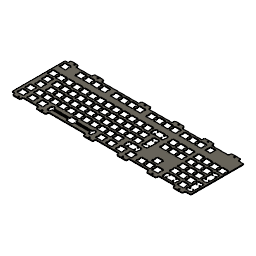
Plate (Autodesk Fusion 360 design; units mm, degrees)
part number: 2026-01-24-23-38-07-205
Autodesk Fusion 360 part; units mm, degrees
(part 1 of 3)
sketch "Sketch2" plane through (0, 0, 0) normal (0, 0, 1) x (1, 0, 0)
  line L0 (432.82, 128.316) -> (432.82, 0.1902)
  line L1 (0.0951, 0.1902) -> (0.0951, 128.316)
  line L2 (126.263, 19.0169) -> (126.263, 18.0165)
  line L3 (126.263, 18.0165) -> (125.462, 18.0165)
  line L4 (125.462, 18.0165) -> (125.462, 14.9173)
  line L5 (125.462, 14.9173) -> (126.263, 14.9173)
  line L6 (126.263, 14.9173) -> (126.263, 14.3164)
  line L7 (126.263, 14.3164) -> (86.6373, 14.3164)
  line L8 (86.6373, 14.3164) -> (86.6373, 17.5466)
  line L9 (86.6373, 17.5466) -> (84.9119, 17.5466)
  line L10 (84.9119, 17.5466) -> (84.9119, 18.4671)
  line L11 (84.9119, 18.4671) -> (81.613, 18.4671)
  line L12 (81.613, 18.4671) -> (81.613, 17.5466)
  line L13 (81.613, 17.5466) -> (79.8876, 17.5466)
  line L14 (79.8876, 17.5466) -> (79.8876, 14.3164)
  line L15 (79.8876, 14.3164) -> (79.0621, 14.3164)
  line L16 (79.0621, 14.3164) -> (79.0621, 11.5163)
  line L17 (79.0621, 11.5163) -> (79.8876, 11.5163)
  line L18 (79.8876, 11.5163) -> (79.8876, 5.2462)
  line L19 (79.8876, 5.2462) -> (81.613, 5.2462)
  line L20 (81.613, 5.2462) -> (81.613, 4.2664)
  line L21 (81.613, 4.2664) -> (84.9119, 4.2664)
  line L22 (84.9119, 4.2664) -> (84.9119, 5.2462)
  line L23 (84.9119, 5.2462) -> (86.6373, 5.2462)
  line L24 (86.6373, 5.2462) -> (86.6373, 9.7166)
  line L25 (86.6373, 9.7166) -> (126.263, 9.7166)
  line L26 (126.263, 9.7166) -> (126.263, 9.1171)
  line L27 (126.263, 9.1171) -> (125.462, 9.1171)
  line L28 (125.462, 9.1171) -> (125.462, 6.0165)
  line L29 (125.462, 6.0165) -> (126.263, 6.0165)
  line L30 (126.263, 6.0165) -> (126.263, 5.0161)
  line L31 (126.263, 5.0161) -> (140.262, 5.0161)
  line L32 (140.262, 5.0161) -> (140.262, 6.0165)
  line L33 (140.262, 6.0165) -> (141.063, 6.0165)
  line L34 (141.063, 6.0165) -> (141.063, 9.1171)
  line L35 (141.063, 9.1171) -> (140.262, 9.1171)
  line L36 (140.262, 9.1171) -> (140.262, 9.7166)
  line L37 (140.262, 9.7166) -> (179.888, 9.7166)
  line L38 (179.888, 9.7166) -> (179.888, 5.2462)
  line L39 (179.888, 5.2462) -> (181.613, 5.2462)
  line L40 (181.613, 5.2462) -> (181.613, 4.2664)
  line L41 (181.613, 4.2664) -> (184.912, 4.2664)
  line L42 (184.912, 4.2664) -> (184.912, 5.2462)
  line L43 (184.912, 5.2462) -> (186.637, 5.2462)
  line L44 (186.637, 5.2462) -> (186.637, 11.5163)
  line L45 (186.637, 11.5163) -> (187.463, 11.5163)
  line L46 (187.463, 11.5163) -> (187.463, 14.3164)
  line L47 (187.463, 14.3164) -> (186.637, 14.3164)
  line L48 (186.637, 14.3164) -> (186.637, 17.5466)
  line L49 (186.637, 17.5466) -> (184.912, 17.5466)
  line L50 (184.912, 17.5466) -> (184.912, 18.4671)
  line L51 (184.912, 18.4671) -> (181.613, 18.4671)
  line L52 (181.613, 18.4671) -> (181.613, 17.5466)
  line L53 (181.613, 17.5466) -> (179.888, 17.5466)
  line L54 (179.888, 17.5466) -> (179.888, 14.3164)
  line L55 (179.888, 14.3164) -> (140.262, 14.3164)
  line L56 (140.262, 14.3164) -> (140.262, 14.9173)
  line L57 (140.262, 14.9173) -> (141.063, 14.9173)
  line L58 (141.063, 14.9173) -> (141.063, 18.0165)
  line L59 (141.063, 18.0165) -> (140.262, 18.0165)
  line L60 (140.262, 18.0165) -> (140.262, 19.0169)
  line L61 (140.262, 19.0169) -> (126.263, 19.0169)
  line L62 (366.769, 19.0169) -> (366.769, 18.0165)
  line L63 (366.769, 18.0165) -> (365.968, 18.0165)
  line L64 (365.968, 18.0165) -> (365.968, 14.9173)
  line L65 (365.968, 14.9173) -> (366.769, 14.9173)
  line L66 (366.769, 14.9173) -> (366.769, 14.3164)
  line L67 (366.769, 14.3164) -> (365.245, 14.3164)
  line L68 (365.245, 14.3164) -> (365.245, 17.5466)
  line L69 (365.245, 17.5466) -> (363.52, 17.5466)
  line L70 (363.52, 17.5466) -> (363.52, 18.4671)
  line L71 (363.52, 18.4671) -> (360.218, 18.4671)
  line L72 (360.218, 18.4671) -> (360.218, 17.5466)
  line L73 (360.218, 17.5466) -> (358.493, 17.5466)
  line L74 (358.493, 17.5466) -> (358.493, 14.3164)
  line L75 (358.493, 14.3164) -> (357.671, 14.3164)
  line L76 (357.671, 14.3164) -> (357.671, 11.5163)
  line L77 (357.671, 11.5163) -> (358.493, 11.5163)
  line L78 (358.493, 11.5163) -> (358.493, 5.2462)
  line L79 (358.493, 5.2462) -> (360.218, 5.2462)
  line L80 (360.218, 5.2462) -> (360.218, 4.2664)
  line L81 (360.218, 4.2664) -> (363.52, 4.2664)
  line L82 (363.52, 4.2664) -> (363.52, 5.2462)
  line L83 (363.52, 5.2462) -> (365.245, 5.2462)
  line L84 (365.245, 5.2462) -> (365.245, 9.7166)
  line L85 (365.245, 9.7166) -> (366.769, 9.7166)
  line L86 (366.769, 9.7166) -> (366.769, 9.1171)
  line L87 (366.769, 9.1171) -> (365.968, 9.1171)
  line L88 (365.968, 9.1171) -> (365.968, 6.0165)
  line L89 (365.968, 6.0165) -> (366.769, 6.0165)
  line L90 (366.769, 6.0165) -> (366.769, 5.0161)
  line L91 (366.769, 5.0161) -> (380.771, 5.0161)
  line L92 (380.771, 5.0161) -> (380.771, 6.0165)
  line L93 (380.771, 6.0165) -> (381.568, 6.0165)
  line L94 (381.568, 6.0165) -> (381.568, 9.1171)
  line L95 (381.568, 9.1171) -> (380.771, 9.1171)
  line L96 (380.771, 9.1171) -> (380.771, 9.7166)
  line L97 (380.771, 9.7166) -> (382.295, 9.7166)
  line L98 (382.295, 9.7166) -> (382.295, 5.2462)
  line L99 (382.295, 5.2462) -> (384.02, 5.2462)
  line L100 (384.02, 5.2462) -> (384.02, 4.2664)
  line L101 (384.02, 4.2664) -> (387.318, 4.2664)
  line L102 (387.318, 4.2664) -> (387.318, 5.2462)
  line L103 (387.318, 5.2462) -> (389.043, 5.2462)
  line L104 (389.043, 5.2462) -> (389.043, 11.5163)
  line L105 (389.043, 11.5163) -> (389.869, 11.5163)
  line L106 (389.869, 11.5163) -> (389.869, 14.3164)
  line L107 (389.869, 14.3164) -> (389.043, 14.3164)
  line L108 (389.043, 14.3164) -> (389.043, 17.5466)
  line L109 (389.043, 17.5466) -> (387.318, 17.5466)
  line L110 (387.318, 17.5466) -> (387.318, 18.4671)
  line L111 (387.318, 18.4671) -> (384.02, 18.4671)
  line L112 (384.02, 18.4671) -> (384.02, 17.5466)
  line L113 (384.02, 17.5466) -> (382.295, 17.5466)
  line L114 (382.295, 17.5466) -> (382.295, 14.3164)
  line L115 (382.295, 14.3164) -> (380.771, 14.3164)
  line L116 (380.771, 14.3164) -> (380.771, 14.9173)
  line L117 (380.771, 14.9173) -> (381.568, 14.9173)
  line L118 (381.568, 14.9173) -> (381.568, 18.0165)
  line L119 (381.568, 18.0165) -> (380.771, 18.0165)
  line L120 (380.771, 18.0165) -> (380.771, 19.0169)
  line L121 (380.771, 19.0169) -> (366.769, 19.0169)
  line L122 (7.2003, 19.0169) -> (7.2003, 18.0165)
  line L123 (7.2003, 18.0165) -> (6.401, 18.0165)
  line L124 (6.401, 18.0165) -> (6.401, 14.9173)
  line L125 (6.401, 14.9173) -> (7.2003, 14.9173)
  line L126 (7.2003, 14.9173) -> (7.2003, 9.1171)
  line L127 (7.2003, 9.1171) -> (6.401, 9.1171)
  line L128 (6.401, 9.1171) -> (6.401, 6.0165)
  line L129 (6.401, 6.0165) -> (7.2003, 6.0165)
  line L130 (7.2003, 6.0165) -> (7.2003, 5.0161)
  line L131 (7.2003, 5.0161) -> (21.2011, 5.0161)
  line L132 (21.2011, 5.0161) -> (21.2011, 6.0165)
  line L133 (21.2011, 6.0165) -> (22.0004, 6.0165)
  line L134 (22.0004, 6.0165) -> (22.0004, 9.1171)
  line L135 (22.0004, 9.1171) -> (21.2011, 9.1171)
  line L136 (21.2011, 9.1171) -> (21.2011, 14.9173)
  line L137 (21.2011, 14.9173) -> (22.0004, 14.9173)
  line L138 (22.0004, 14.9173) -> (22.0004, 18.0165)
  line L139 (22.0004, 18.0165) -> (21.2011, 18.0165)
  line L140 (21.2011, 18.0165) -> (21.2011, 19.0169)
  line L141 (21.2011, 19.0169) -> (7.2003, 19.0169)
  line L142 (31.0128, 19.0169) -> (31.0128, 18.0165)
  line L143 (31.0128, 18.0165) -> (30.2121, 18.0165)
  line L144 (30.2121, 18.0165) -> (30.2121, 14.9173)
  line L145 (30.2121, 14.9173) -> (31.0128, 14.9173)
  line L146 (31.0128, 14.9173) -> (31.0128, 9.1171)
  line L147 (31.0128, 9.1171) -> (30.2121, 9.1171)
  line L148 (30.2121, 9.1171) -> (30.2121, 6.0165)
  line L149 (30.2121, 6.0165) -> (31.0128, 6.0165)
  line L150 (31.0128, 6.0165) -> (31.0128, 5.0161)
  line L151 (31.0128, 5.0161) -> (45.0123, 5.0161)
  line L152 (45.0123, 5.0161) -> (45.0123, 6.0165)
  line L153 (45.0123, 6.0165) -> (45.8128, 6.0165)
  line L154 (45.8128, 6.0165) -> (45.8128, 9.1171)
  line L155 (45.8128, 9.1171) -> (45.0123, 9.1171)
  line L156 (45.0123, 9.1171) -> (45.0123, 14.9173)
  line L157 (45.0123, 14.9173) -> (45.8128, 14.9173)
  line L158 (45.8128, 14.9173) -> (45.8128, 18.0165)
  line L159 (45.8128, 18.0165) -> (45.0123, 18.0165)
  line L160 (45.0123, 18.0165) -> (45.0123, 19.0169)
  line L161 (45.0123, 19.0169) -> (31.0128, 19.0169)
  line L162 (54.8252, 19.0169) -> (54.8252, 18.0165)
  line L163 (54.8252, 18.0165) -> (54.0262, 18.0165)
  line L164 (54.0262, 18.0165) -> (54.0262, 14.9173)
  line L165 (54.0262, 14.9173) -> (54.8252, 14.9173)
  line L166 (54.8252, 14.9173) -> (54.8252, 9.1171)
  line L167 (54.8252, 9.1171) -> (54.0262, 9.1171)
  line L168 (54.0262, 9.1171) -> (54.0262, 6.0165)
  line L169 (54.0262, 6.0165) -> (54.8252, 6.0165)
  line L170 (54.8252, 6.0165) -> (54.8252, 5.0161)
  line L171 (54.8252, 5.0161) -> (68.8262, 5.0161)
  line L172 (68.8262, 5.0161) -> (68.8262, 6.0165)
  line L173 (68.8262, 6.0165) -> (69.6253, 6.0165)
  line L174 (69.6253, 6.0165) -> (69.6253, 9.1171)
  line L175 (69.6253, 9.1171) -> (68.8262, 9.1171)
  line L176 (68.8262, 9.1171) -> (68.8262, 14.9173)
  line L177 (68.8262, 14.9173) -> (69.6253, 14.9173)
  line L178 (69.6253, 14.9173) -> (69.6253, 18.0165)
  line L179 (69.6253, 18.0165) -> (68.8262, 18.0165)
  line L180 (68.8262, 18.0165) -> (68.8262, 19.0169)
  line L181 (68.8262, 19.0169) -> (54.8252, 19.0169)
  line L182 (197.7, 19.0169) -> (197.7, 18.0165)
  line L183 (197.7, 18.0165) -> (196.901, 18.0165)
  line L184 (196.901, 18.0165) -> (196.901, 14.9173)
  line L185 (196.901, 14.9173) -> (197.7, 14.9173)
  line L186 (197.7, 14.9173) -> (197.7, 9.1171)
  line L187 (197.7, 9.1171) -> (196.901, 9.1171)
  line L188 (196.901, 9.1171) -> (196.901, 6.0165)
  line L189 (196.901, 6.0165) -> (197.7, 6.0165)
  line L190 (197.7, 6.0165) -> (197.7, 5.0161)
  line L191 (197.7, 5.0161) -> (211.701, 5.0161)
  line L192 (211.701, 5.0161) -> (211.701, 6.0165)
  line L193 (211.701, 6.0165) -> (212.5, 6.0165)
  line L194 (212.5, 6.0165) -> (212.5, 9.1171)
  line L195 (212.5, 9.1171) -> (211.701, 9.1171)
  line L196 (211.701, 9.1171) -> (211.701, 14.9173)
  line L197 (211.701, 14.9173) -> (212.5, 14.9173)
  line L198 (212.5, 14.9173) -> (212.5, 18.0165)
  line L199 (212.5, 18.0165) -> (211.701, 18.0165)
  line L200 (211.701, 18.0165) -> (211.701, 19.0169)
  line L201 (211.701, 19.0169) -> (197.7, 19.0169)
  line L202 (221.513, 19.0169) -> (221.513, 18.0165)
  line L203 (221.513, 18.0165) -> (220.712, 18.0165)
  line L204 (220.712, 18.0165) -> (220.712, 14.9173)
  line L205 (220.712, 14.9173) -> (221.513, 14.9173)
  line L206 (221.513, 14.9173) -> (221.513, 9.1171)
  line L207 (221.513, 9.1171) -> (220.712, 9.1171)
  line L208 (220.712, 9.1171) -> (220.712, 6.0165)
  line L209 (220.712, 6.0165) -> (221.513, 6.0165)
  line L210 (221.513, 6.0165) -> (221.513, 5.0161)
  line L211 (221.513, 5.0161) -> (235.512, 5.0161)
  line L212 (235.512, 5.0161) -> (235.512, 6.0165)
  line L213 (235.512, 6.0165) -> (236.313, 6.0165)
  line L214 (236.313, 6.0165) -> (236.313, 9.1171)
  line L215 (236.313, 9.1171) -> (235.512, 9.1171)
  line L216 (235.512, 9.1171) -> (235.512, 14.9173)
  line L217 (235.512, 14.9173) -> (236.313, 14.9173)
  line L218 (236.313, 14.9173) -> (236.313, 18.0165)
  line L219 (236.313, 18.0165) -> (235.512, 18.0165)
  line L220 (235.512, 18.0165) -> (235.512, 19.0169)
  line L221 (235.512, 19.0169) -> (221.513, 19.0169)
  line L222 (245.325, 19.0169) -> (245.325, 18.0165)
  line L223 (245.325, 18.0165) -> (244.526, 18.0165)
  line L224 (244.526, 18.0165) -> (244.526, 14.9173)
  line L225 (244.526, 14.9173) -> (245.325, 14.9173)
  line L226 (245.325, 14.9173) -> (245.325, 9.1171)
  line L227 (245.325, 9.1171) -> (244.526, 9.1171)
  line L228 (244.526, 9.1171) -> (244.526, 6.0165)
  line L229 (244.526, 6.0165) -> (245.325, 6.0165)
  line L230 (245.325, 6.0165) -> (245.325, 5.0161)
  line L231 (245.325, 5.0161) -> (259.326, 5.0161)
  line L232 (259.326, 5.0161) -> (259.326, 6.0165)
  line L233 (259.326, 6.0165) -> (260.125, 6.0165)
  line L234 (260.125, 6.0165) -> (260.125, 9.1171)
  line L235 (260.125, 9.1171) -> (259.326, 9.1171)
  line L236 (259.326, 9.1171) -> (259.326, 14.9173)
  line L237 (259.326, 14.9173) -> (260.125, 14.9173)
  line L238 (260.125, 14.9173) -> (260.125, 18.0165)
  line L239 (260.125, 18.0165) -> (259.326, 18.0165)
  line L240 (259.326, 18.0165) -> (259.326, 19.0169)
  line L241 (259.326, 19.0169) -> (245.325, 19.0169)
  line L242 (269.138, 19.0169) -> (269.138, 18.0165)
  line L243 (269.138, 18.0165) -> (268.337, 18.0165)
  line L244 (268.337, 18.0165) -> (268.337, 14.9173)
  line L245 (268.337, 14.9173) -> (269.138, 14.9173)
  line L246 (269.138, 14.9173) -> (269.138, 9.1171)
  line L247 (269.138, 9.1171) -> (268.337, 9.1171)
  line L248 (268.337, 9.1171) -> (268.337, 6.0165)
  line L249 (268.337, 6.0165) -> (269.138, 6.0165)
  line L250 (269.138, 6.0165) -> (269.138, 5.0161)
  line L251 (269.138, 5.0161) -> (283.137, 5.0161)
  line L252 (283.137, 5.0161) -> (283.137, 6.0165)
  line L253 (283.137, 6.0165) -> (283.938, 6.0165)
  line L254 (283.938, 6.0165) -> (283.938, 9.1171)
  line L255 (283.938, 9.1171) -> (283.137, 9.1171)
  line L256 (283.137, 9.1171) -> (283.137, 14.9173)
  line L257 (283.137, 14.9173) -> (283.938, 14.9173)
  line L258 (283.938, 14.9173) -> (283.938, 18.0165)
  line L259 (283.938, 18.0165) -> (283.137, 18.0165)
  line L260 (283.137, 18.0165) -> (283.137, 19.0169)
  line L261 (283.137, 19.0169) -> (269.138, 19.0169)
  line L262 (295.331, 19.0169) -> (295.331, 18.0165)
  line L263 (295.331, 18.0165) -> (294.531, 18.0165)
  line L264 (294.531, 18.0165) -> (294.531, 14.9173)
  line L265 (294.531, 14.9173) -> (295.331, 14.9173)
  line L266 (295.331, 14.9173) -> (295.331, 9.1171)
  line L267 (295.331, 9.1171) -> (294.531, 9.1171)
  line L268 (294.531, 9.1171) -> (294.531, 6.0165)
  line L269 (294.531, 6.0165) -> (295.331, 6.0165)
  line L270 (295.331, 6.0165) -> (295.331, 5.0161)
  line L271 (295.331, 5.0161) -> (309.331, 5.0161)
  line L272 (309.331, 5.0161) -> (309.331, 6.0165)
  line L273 (309.331, 6.0165) -> (310.132, 6.0165)
  line L274 (310.132, 6.0165) -> (310.132, 9.1171)
  line L275 (310.132, 9.1171) -> (309.331, 9.1171)
  line L276 (309.331, 9.1171) -> (309.331, 14.9173)
  line L277 (309.331, 14.9173) -> (310.132, 14.9173)
  line L278 (310.132, 14.9173) -> (310.132, 18.0165)
  line L279 (310.132, 18.0165) -> (309.331, 18.0165)
  line L280 (309.331, 18.0165) -> (309.331, 19.0169)
  line L281 (309.331, 19.0169) -> (295.331, 19.0169)
  line L282 (314.381, 19.0169) -> (314.381, 18.0165)
  line L283 (314.381, 18.0165) -> (313.581, 18.0165)
  line L284 (313.581, 18.0165) -> (313.581, 14.9173)
  line L285 (313.581, 14.9173) -> (314.381, 14.9173)
  line L286 (314.381, 14.9173) -> (314.381, 9.1171)
  line L287 (314.381, 9.1171) -> (313.581, 9.1171)
  line L288 (313.581, 9.1171) -> (313.581, 6.0165)
  line L289 (313.581, 6.0165) -> (314.381, 6.0165)
  line L290 (314.381, 6.0165) -> (314.381, 5.0161)
  line L291 (314.381, 5.0161) -> (328.381, 5.0161)
  line L292 (328.381, 5.0161) -> (328.381, 6.0165)
  line L293 (328.381, 6.0165) -> (329.182, 6.0165)
  line L294 (329.182, 6.0165) -> (329.182, 9.1171)
  line L295 (329.182, 9.1171) -> (328.381, 9.1171)
  line L296 (328.381, 9.1171) -> (328.381, 14.9173)
  line L297 (328.381, 14.9173) -> (329.182, 14.9173)
  line L298 (329.182, 14.9173) -> (329.182, 18.0165)
  line L299 (329.182, 18.0165) -> (328.381, 18.0165)
  line L300 (328.381, 18.0165) -> (328.381, 19.0169)
  line L301 (328.381, 19.0169) -> (314.381, 19.0169)
  line L302 (333.431, 19.0169) -> (333.431, 18.0165)
  line L303 (333.431, 18.0165) -> (332.631, 18.0165)
  line L304 (332.631, 18.0165) -> (332.631, 14.9173)
  line L305 (332.631, 14.9173) -> (333.431, 14.9173)
  line L306 (333.431, 14.9173) -> (333.431, 9.1171)
  line L307 (333.431, 9.1171) -> (332.631, 9.1171)
  line L308 (332.631, 9.1171) -> (332.631, 6.0165)
  line L309 (332.631, 6.0165) -> (333.431, 6.0165)
  line L310 (333.431, 6.0165) -> (333.431, 5.0161)
  line L311 (333.431, 5.0161) -> (347.431, 5.0161)
  line L312 (347.431, 5.0161) -> (347.431, 6.0165)
  line L313 (347.431, 6.0165) -> (348.232, 6.0165)
  line L314 (348.232, 6.0165) -> (348.232, 9.1171)
  line L315 (348.232, 9.1171) -> (347.431, 9.1171)
  line L316 (347.431, 9.1171) -> (347.431, 14.9173)
  line L317 (347.431, 14.9173) -> (348.232, 14.9173)
  line L318 (348.232, 14.9173) -> (348.232, 18.0165)
  line L319 (348.232, 18.0165) -> (347.431, 18.0165)
  line L320 (347.431, 18.0165) -> (347.431, 19.0169)
  line L321 (347.431, 19.0169) -> (333.431, 19.0169)
  line L322 (395.344, 19.0169) -> (395.344, 18.0165)
  line L323 (395.344, 18.0165) -> (394.543, 18.0165)
  line L324 (394.543, 18.0165) -> (394.543, 14.9173)
  line L325 (394.543, 14.9173) -> (395.344, 14.9173)
  line L326 (395.344, 14.9173) -> (395.344, 9.1171)
  line L327 (395.344, 9.1171) -> (394.543, 9.1171)
  line L328 (394.543, 9.1171) -> (394.543, 6.0165)
  line L329 (394.543, 6.0165) -> (395.344, 6.0165)
  line L330 (395.344, 6.0165) -> (395.344, 5.0161)
  line L331 (395.344, 5.0161) -> (409.346, 5.0161)
  line L332 (409.346, 5.0161) -> (409.346, 6.0165)
  line L333 (409.346, 6.0165) -> (410.143, 6.0165)
  line L334 (410.143, 6.0165) -> (410.143, 9.1171)
  line L335 (410.143, 9.1171) -> (409.346, 9.1171)
  line L336 (409.346, 9.1171) -> (409.346, 14.9173)
  line L337 (409.346, 14.9173) -> (410.143, 14.9173)
  line L338 (410.143, 14.9173) -> (410.143, 18.0165)
  line L339 (410.143, 18.0165) -> (409.346, 18.0165)
  line L340 (409.346, 18.0165) -> (409.346, 19.0169)
  line L341 (409.346, 19.0169) -> (395.344, 19.0169)
  line L342 (420.896, 37.641) -> (420.896, 36.8169)
  line L343 (420.896, 36.8169) -> (414.623, 36.8169)
  line L344 (414.623, 36.8169) -> (414.623, 35.0918)
  line L345 (414.623, 35.0918) -> (413.646, 35.0918)
  line L346 (413.646, 35.0918) -> (413.646, 31.7913)
  line L347 (413.646, 31.7913) -> (414.623, 31.7913)
  line L348 (414.623, 31.7913) -> (414.623, 30.0661)
  line L349 (414.623, 30.0661) -> (419.093, 30.0661)
  line L350 (419.093, 30.0661) -> (419.093, 28.5419)
  line L351 (419.093, 28.5419) -> (418.497, 28.5419)
  line L352 (418.497, 28.5419) -> (418.497, 29.3412)
  line L353 (418.497, 29.3412) -> (415.396, 29.3412)
  line L354 (415.396, 29.3412) -> (415.396, 28.5419)
  line L355 (415.396, 28.5419) -> (414.394, 28.5419)
  line L356 (414.394, 28.5419) -> (414.394, 14.5411)
  line L357 (414.394, 14.5411) -> (415.396, 14.5411)
  line L358 (415.396, 14.5411) -> (415.396, 13.7418)
  line L359 (415.396, 13.7418) -> (418.497, 13.7418)
  line L360 (418.497, 13.7418) -> (418.497, 14.5411)
  line L361 (418.497, 14.5411) -> (419.093, 14.5411)
  line L362 (419.093, 14.5411) -> (419.093, 13.0169)
  line L363 (419.093, 13.0169) -> (414.623, 13.0169)
  line L364 (414.623, 13.0169) -> (414.623, 11.2916)
  line L365 (414.623, 11.2916) -> (413.646, 11.2916)
  line L366 (413.646, 11.2916) -> (413.646, 7.9912)
  line L367 (413.646, 7.9912) -> (414.623, 7.9912)
  line L368 (414.623, 7.9912) -> (414.623, 6.2659)
  line L369 (414.623, 6.2659) -> (420.896, 6.2659)
  line L370 (420.896, 6.2659) -> (420.896, 5.4419)
  line L371 (420.896, 5.4419) -> (423.693, 5.4419)
  line L372 (423.693, 5.4419) -> (423.693, 6.2659)
  line L373 (423.693, 6.2659) -> (426.925, 6.2659)
  line L374 (426.925, 6.2659) -> (426.925, 7.9912)
  line L375 (426.925, 7.9912) -> (427.845, 7.9912)
  line L376 (427.845, 7.9912) -> (427.845, 11.2916)
  line L377 (427.845, 11.2916) -> (426.925, 11.2916)
  line L378 (426.925, 11.2916) -> (426.925, 13.0169)
  line L379 (426.925, 13.0169) -> (423.693, 13.0169)
  line L380 (423.693, 13.0169) -> (423.693, 14.5411)
  line L381 (423.693, 14.5411) -> (424.293, 14.5411)
  line L382 (424.293, 14.5411) -> (424.293, 13.7418)
  line L383 (424.293, 13.7418) -> (427.394, 13.7418)
  line L384 (427.394, 13.7418) -> (427.394, 14.5411)
  line L385 (427.394, 14.5411) -> (428.396, 14.5411)
  line L386 (428.396, 14.5411) -> (428.396, 28.5419)
  line L387 (428.396, 28.5419) -> (427.394, 28.5419)
  line L388 (427.394, 28.5419) -> (427.394, 29.3412)
  line L389 (427.394, 29.3412) -> (424.293, 29.3412)
  line L390 (424.293, 29.3412) -> (424.293, 28.5419)
  line L391 (424.293, 28.5419) -> (423.693, 28.5419)
  line L392 (423.693, 28.5419) -> (423.693, 30.0661)
  line L393 (423.693, 30.0661) -> (426.925, 30.0661)
  line L394 (426.925, 30.0661) -> (426.925, 31.7913)
  line L395 (426.925, 31.7913) -> (427.845, 31.7913)
  line L396 (427.845, 31.7913) -> (427.845, 35.0918)
  line L397 (427.845, 35.0918) -> (426.925, 35.0918)
  line L398 (426.925, 35.0918) -> (426.925, 36.8169)
  line L399 (426.925, 36.8169) -> (423.693, 36.8169)
  line L400 (423.693, 36.8169) -> (423.693, 37.641)
  line L401 (423.693, 37.641) -> (420.896, 37.641)
  line L402 (254.849, 38.0668) -> (254.849, 37.0664)
  line L403 (254.849, 37.0664) -> (254.051, 37.0664)
  line L404 (254.051, 37.0664) -> (254.051, 33.9673)
  line L405 (254.051, 33.9673) -> (254.849, 33.9673)
  line L406 (254.849, 33.9673) -> (254.849, 33.3664)
  line L407 (254.849, 33.3664) -> (253.326, 33.3664)
  line L408 (253.326, 33.3664) -> (253.326, 36.5965)
  line L409 (253.326, 36.5965) -> (251.599, 36.5965)
  line L410 (251.599, 36.5965) -> (251.599, 37.5172)
  line L411 (251.599, 37.5172) -> (248.301, 37.5172)
  line L412 (248.301, 37.5172) -> (248.301, 36.5965)
  line L413 (248.301, 36.5965) -> (246.575, 36.5965)
  line L414 (246.575, 36.5965) -> (246.575, 33.3664)
  line L415 (246.575, 33.3664) -> (245.751, 33.3664)
  line L416 (245.751, 33.3664) -> (245.751, 30.5663)
  line L417 (245.751, 30.5663) -> (246.575, 30.5663)
  line L418 (246.575, 30.5663) -> (246.575, 24.2962)
  line L419 (246.575, 24.2962) -> (248.301, 24.2962)
  line L420 (248.301, 24.2962) -> (248.301, 23.3164)
  line L421 (248.301, 23.3164) -> (251.599, 23.3164)
  line L422 (251.599, 23.3164) -> (251.599, 24.2962)
  line L423 (251.599, 24.2962) -> (253.326, 24.2962)
  line L424 (253.326, 24.2962) -> (253.326, 28.7666)
  line L425 (253.326, 28.7666) -> (254.849, 28.7666)
  line L426 (254.849, 28.7666) -> (254.849, 28.1671)
  line L427 (254.849, 28.1671) -> (254.051, 28.1671)
  line L428 (254.051, 28.1671) -> (254.051, 25.0665)
  line L429 (254.051, 25.0665) -> (254.849, 25.0665)
  line L430 (254.849, 25.0665) -> (254.849, 24.0661)
  line L431 (254.849, 24.0661) -> (268.851, 24.0661)
  line L432 (268.851, 24.0661) -> (268.851, 25.0665)
  line L433 (268.851, 25.0665) -> (269.65, 25.0665)
  line L434 (269.65, 25.0665) -> (269.65, 28.1671)
  line L435 (269.65, 28.1671) -> (268.851, 28.1671)
  line L436 (268.851, 28.1671) -> (268.851, 28.7666)
  line L437 (268.851, 28.7666) -> (270.375, 28.7666)
  line L438 (270.375, 28.7666) -> (270.375, 24.2962)
  line L439 (270.375, 24.2962) -> (272.101, 24.2962)
  line L440 (272.101, 24.2962) -> (272.101, 23.3164)
  line L441 (272.101, 23.3164) -> (275.401, 23.3164)
  line L442 (275.401, 23.3164) -> (275.401, 24.2962)
  line L443 (275.401, 24.2962) -> (277.125, 24.2962)
  line L444 (277.125, 24.2962) -> (277.125, 30.5663)
  line L445 (277.125, 30.5663) -> (277.95, 30.5663)
  line L446 (277.95, 30.5663) -> (277.95, 33.3664)
  line L447 (277.95, 33.3664) -> (277.125, 33.3664)
  line L448 (277.125, 33.3664) -> (277.125, 36.5965)
  line L449 (277.125, 36.5965) -> (275.401, 36.5965)
  line L450 (275.401, 36.5965) -> (275.401, 37.5172)
  line L451 (275.401, 37.5172) -> (272.101, 37.5172)
  line L452 (272.101, 37.5172) -> (272.101, 36.5965)
  line L453 (272.101, 36.5965) -> (270.375, 36.5965)
  line L454 (270.375, 36.5965) -> (270.375, 33.3664)
  line L455 (270.375, 33.3664) -> (268.851, 33.3664)
  line L456 (268.851, 33.3664) -> (268.851, 33.9673)
  line L457 (268.851, 33.9673) -> (269.65, 33.9673)
  line L458 (269.65, 33.9673) -> (269.65, 37.0664)
  line L459 (269.65, 37.0664) -> (268.851, 37.0664)
  line L460 (268.851, 37.0664) -> (268.851, 38.0668)
  line L461 (268.851, 38.0668) -> (254.849, 38.0668)
  line L462 (7.2003, 38.0668) -> (7.2003, 37.0664)
  line L463 (7.2003, 37.0664) -> (6.401, 37.0664)
  line L464 (6.401, 37.0664) -> (6.401, 33.9673)
  line L465 (6.401, 33.9673) -> (7.2003, 33.9673)
  line L466 (7.2003, 33.9673) -> (7.2003, 28.1671)
  line L467 (7.2003, 28.1671) -> (6.401, 28.1671)
  line L468 (6.401, 28.1671) -> (6.401, 25.0665)
  line L469 (6.401, 25.0665) -> (7.2003, 25.0665)
  line L470 (7.2003, 25.0665) -> (7.2003, 24.0661)
  line L471 (7.2003, 24.0661) -> (21.2011, 24.0661)
  line L472 (21.2011, 24.0661) -> (21.2011, 25.0665)
  line L473 (21.2011, 25.0665) -> (22.0004, 25.0665)
  line L474 (22.0004, 25.0665) -> (22.0004, 28.1671)
  line L475 (22.0004, 28.1671) -> (21.2011, 28.1671)
  line L476 (21.2011, 28.1671) -> (21.2011, 33.9673)
  line L477 (21.2011, 33.9673) -> (22.0004, 33.9673)
  line L478 (22.0004, 33.9673) -> (22.0004, 37.0664)
  line L479 (22.0004, 37.0664) -> (21.2011, 37.0664)
  line L480 (21.2011, 37.0664) -> (21.2011, 38.0668)
  line L481 (21.2011, 38.0668) -> (7.2003, 38.0668)
  line L482 (28.6315, 38.0668) -> (28.6315, 37.0664)
  line L483 (28.6315, 37.0664) -> (27.8309, 37.0664)
  line L484 (27.8309, 37.0664) -> (27.8309, 33.9673)
  line L485 (27.8309, 33.9673) -> (28.6315, 33.9673)
  line L486 (28.6315, 33.9673) -> (28.6315, 28.1671)
  line L487 (28.6315, 28.1671) -> (27.8309, 28.1671)
  line L488 (27.8309, 28.1671) -> (27.8309, 25.0665)
  line L489 (27.8309, 25.0665) -> (28.6315, 25.0665)
  line L490 (28.6315, 25.0665) -> (28.6315, 24.0661)
  line L491 (28.6315, 24.0661) -> (42.6311, 24.0661)
  line L492 (42.6311, 24.0661) -> (42.6311, 25.0665)
  line L493 (42.6311, 25.0665) -> (43.4315, 25.0665)
  line L494 (43.4315, 25.0665) -> (43.4315, 28.1671)
  line L495 (43.4315, 28.1671) -> (42.6311, 28.1671)
  line L496 (42.6311, 28.1671) -> (42.6311, 33.9673)
  line L497 (42.6311, 33.9673) -> (43.4315, 33.9673)
  line L498 (43.4315, 33.9673) -> (43.4315, 37.0664)
  line L499 (43.4315, 37.0664) -> (42.6311, 37.0664)
  line L500 (42.6311, 37.0664) -> (42.6311, 38.0668)
  line L501 (42.6311, 38.0668) -> (28.6315, 38.0668)
  line L502 (47.6814, 38.0668) -> (47.6814, 37.0664)
  line L503 (47.6814, 37.0664) -> (46.881, 37.0664)
  line L504 (46.881, 37.0664) -> (46.881, 33.9673)
  line L505 (46.881, 33.9673) -> (47.6814, 33.9673)
  line L506 (47.6814, 33.9673) -> (47.6814, 28.1671)
  line L507 (47.6814, 28.1671) -> (46.881, 28.1671)
  line L508 (46.881, 28.1671) -> (46.881, 25.0665)
  line L509 (46.881, 25.0665) -> (47.6814, 25.0665)
  line L510 (47.6814, 25.0665) -> (47.6814, 24.0661)
  line L511 (47.6814, 24.0661) -> (61.6811, 24.0661)
  line L512 (61.6811, 24.0661) -> (61.6811, 25.0665)
  line L513 (61.6811, 25.0665) -> (62.4815, 25.0665)
  line L514 (62.4815, 25.0665) -> (62.4815, 28.1671)
  line L515 (62.4815, 28.1671) -> (61.6811, 28.1671)
  line L516 (61.6811, 28.1671) -> (61.6811, 33.9673)
  line L517 (61.6811, 33.9673) -> (62.4815, 33.9673)
  line L518 (62.4815, 33.9673) -> (62.4815, 37.0664)
  line L519 (62.4815, 37.0664) -> (61.6811, 37.0664)
  line L520 (61.6811, 37.0664) -> (61.6811, 38.0668)
  line L521 (61.6811, 38.0668) -> (47.6814, 38.0668)
  line L522 (66.7314, 38.0668) -> (66.7314, 37.0664)
  line L523 (66.7314, 37.0664) -> (65.931, 37.0664)
  line L524 (65.931, 37.0664) -> (65.931, 33.9673)
  line L525 (65.931, 33.9673) -> (66.7314, 33.9673)
  line L526 (66.7314, 33.9673) -> (66.7314, 28.1671)
  line L527 (66.7314, 28.1671) -> (65.931, 28.1671)
  line L528 (65.931, 28.1671) -> (65.931, 25.0665)
  line L529 (65.931, 25.0665) -> (66.7314, 25.0665)
  line L530 (66.7314, 25.0665) -> (66.7314, 24.0661)
  line L531 (66.7314, 24.0661) -> (80.7311, 24.0661)
  line L532 (80.7311, 24.0661) -> (80.7311, 25.0665)
  line L533 (80.7311, 25.0665) -> (81.5315, 25.0665)
  line L534 (81.5315, 25.0665) -> (81.5315, 28.1671)
  line L535 (81.5315, 28.1671) -> (80.7311, 28.1671)
  line L536 (80.7311, 28.1671) -> (80.7311, 33.9673)
  line L537 (80.7311, 33.9673) -> (81.5315, 33.9673)
  line L538 (81.5315, 33.9673) -> (81.5315, 37.0664)
  line L539 (81.5315, 37.0664) -> (80.7311, 37.0664)
  line L540 (80.7311, 37.0664) -> (80.7311, 38.0668)
  line L541 (80.7311, 38.0668) -> (66.7314, 38.0668)
  line L542 (85.7814, 38.0668) -> (85.7814, 37.0664)
  line L543 (85.7814, 37.0664) -> (84.981, 37.0664)
  line L544 (84.981, 37.0664) -> (84.981, 33.9673)
  line L545 (84.981, 33.9673) -> (85.7814, 33.9673)
  line L546 (85.7814, 33.9673) -> (85.7814, 28.1671)
  line L547 (85.7814, 28.1671) -> (84.981, 28.1671)
  line L548 (84.981, 28.1671) -> (84.981, 25.0665)
  line L549 (84.981, 25.0665) -> (85.7814, 25.0665)
  line L550 (85.7814, 25.0665) -> (85.7814, 24.0661)
  line L551 (85.7814, 24.0661) -> (99.7811, 24.0661)
  line L552 (99.7811, 24.0661) -> (99.7811, 25.0665)
  line L553 (99.7811, 25.0665) -> (100.582, 25.0665)
  line L554 (100.582, 25.0665) -> (100.582, 28.1671)
  line L555 (100.582, 28.1671) -> (99.7811, 28.1671)
  line L556 (99.7811, 28.1671) -> (99.7811, 33.9673)
  line L557 (99.7811, 33.9673) -> (100.582, 33.9673)
  line L558 (100.582, 33.9673) -> (100.582, 37.0664)
  line L559 (100.582, 37.0664) -> (99.7811, 37.0664)
  line L560 (99.7811, 37.0664) -> (99.7811, 38.0668)
  line L561 (99.7811, 38.0668) -> (85.7814, 38.0668)
  line L562 (104.831, 38.0668) -> (104.831, 37.0664)
  line L563 (104.831, 37.0664) -> (104.031, 37.0664)
  line L564 (104.031, 37.0664) -> (104.031, 33.9673)
  line L565 (104.031, 33.9673) -> (104.831, 33.9673)
  line L566 (104.831, 33.9673) -> (104.831, 28.1671)
  line L567 (104.831, 28.1671) -> (104.031, 28.1671)
  line L568 (104.031, 28.1671) -> (104.031, 25.0665)
  line L569 (104.031, 25.0665) -> (104.831, 25.0665)
  line L570 (104.831, 25.0665) -> (104.831, 24.0661)
  line L571 (104.831, 24.0661) -> (118.831, 24.0661)
  line L572 (118.831, 24.0661) -> (118.831, 25.0665)
  line L573 (118.831, 25.0665) -> (119.632, 25.0665)
  line L574 (119.632, 25.0665) -> (119.632, 28.1671)
  line L575 (119.632, 28.1671) -> (118.831, 28.1671)
  line L576 (118.831, 28.1671) -> (118.831, 33.9673)
  line L577 (118.831, 33.9673) -> (119.632, 33.9673)
  line L578 (119.632, 33.9673) -> (119.632, 37.0664)
  line L579 (119.632, 37.0664) -> (118.831, 37.0664)
  line L580 (118.831, 37.0664) -> (118.831, 38.0668)
  line L581 (118.831, 38.0668) -> (104.831, 38.0668)
  line L582 (123.881, 38.0668) -> (123.881, 37.0664)
  line L583 (123.881, 37.0664) -> (123.081, 37.0664)
  line L584 (123.081, 37.0664) -> (123.081, 33.9673)
  line L585 (123.081, 33.9673) -> (123.881, 33.9673)
  line L586 (123.881, 33.9673) -> (123.881, 28.1671)
  line L587 (123.881, 28.1671) -> (123.081, 28.1671)
  line L588 (123.081, 28.1671) -> (123.081, 25.0665)
  line L589 (123.081, 25.0665) -> (123.881, 25.0665)
  line L590 (123.881, 25.0665) -> (123.881, 24.0661)
  line L591 (123.881, 24.0661) -> (137.881, 24.0661)
  line L592 (137.881, 24.0661) -> (137.881, 25.0665)
  line L593 (137.881, 25.0665) -> (138.682, 25.0665)
  line L594 (138.682, 25.0665) -> (138.682, 28.1671)
  line L595 (138.682, 28.1671) -> (137.881, 28.1671)
  line L596 (137.881, 28.1671) -> (137.881, 33.9673)
  line L597 (137.881, 33.9673) -> (138.682, 33.9673)
  line L598 (138.682, 33.9673) -> (138.682, 37.0664)
  line L599 (138.682, 37.0664) -> (137.881, 37.0664)
  line L600 (137.881, 37.0664) -> (137.881, 38.0668)
  line L601 (137.881, 38.0668) -> (123.881, 38.0668)
  line L602 (142.931, 38.0668) -> (142.931, 37.0664)
  line L603 (142.931, 37.0664) -> (142.131, 37.0664)
  line L604 (142.131, 37.0664) -> (142.131, 33.9673)
  line L605 (142.131, 33.9673) -> (142.931, 33.9673)
  line L606 (142.931, 33.9673) -> (142.931, 28.1671)
  line L607 (142.931, 28.1671) -> (142.131, 28.1671)
  line L608 (142.131, 28.1671) -> (142.131, 25.0665)
  line L609 (142.131, 25.0665) -> (142.931, 25.0665)
  line L610 (142.931, 25.0665) -> (142.931, 24.0661)
  line L611 (142.931, 24.0661) -> (156.931, 24.0661)
  line L612 (156.931, 24.0661) -> (156.931, 25.0665)
  line L613 (156.931, 25.0665) -> (157.732, 25.0665)
  line L614 (157.732, 25.0665) -> (157.732, 28.1671)
  line L615 (157.732, 28.1671) -> (156.931, 28.1671)
  line L616 (156.931, 28.1671) -> (156.931, 33.9673)
  line L617 (156.931, 33.9673) -> (157.732, 33.9673)
  line L618 (157.732, 33.9673) -> (157.732, 37.0664)
  line L619 (157.732, 37.0664) -> (156.931, 37.0664)
  line L620 (156.931, 37.0664) -> (156.931, 38.0668)
  line L621 (156.931, 38.0668) -> (142.931, 38.0668)
  line L622 (161.981, 38.0668) -> (161.981, 37.0664)
  line L623 (161.981, 37.0664) -> (161.181, 37.0664)
  line L624 (161.181, 37.0664) -> (161.181, 33.9673)
  line L625 (161.181, 33.9673) -> (161.981, 33.9673)
  line L626 (161.981, 33.9673) -> (161.981, 28.1671)
  line L627 (161.981, 28.1671) -> (161.181, 28.1671)
  line L628 (161.181, 28.1671) -> (161.181, 25.0665)
  line L629 (161.181, 25.0665) -> (161.981, 25.0665)
  line L630 (161.981, 25.0665) -> (161.981, 24.0661)
  line L631 (161.981, 24.0661) -> (175.981, 24.0661)
  line L632 (175.981, 24.0661) -> (175.981, 25.0665)
  line L633 (175.981, 25.0665) -> (176.782, 25.0665)
  line L634 (176.782, 25.0665) -> (176.782, 28.1671)
  line L635 (176.782, 28.1671) -> (175.981, 28.1671)
  line L636 (175.981, 28.1671) -> (175.981, 33.9673)
  line L637 (175.981, 33.9673) -> (176.782, 33.9673)
  line L638 (176.782, 33.9673) -> (176.782, 37.0664)
  line L639 (176.782, 37.0664) -> (175.981, 37.0664)
  line L640 (175.981, 37.0664) -> (175.981, 38.0668)
  line L641 (175.981, 38.0668) -> (161.981, 38.0668)
  line L642 (181.031, 38.0668) -> (181.031, 37.0664)
  line L643 (181.031, 37.0664) -> (180.231, 37.0664)
  line L644 (180.231, 37.0664) -> (180.231, 33.9673)
  line L645 (180.231, 33.9673) -> (181.031, 33.9673)
  line L646 (181.031, 33.9673) -> (181.031, 28.1671)
  line L647 (181.031, 28.1671) -> (180.231, 28.1671)
  line L648 (180.231, 28.1671) -> (180.231, 25.0665)
  line L649 (180.231, 25.0665) -> (181.031, 25.0665)
  line L650 (181.031, 25.0665) -> (181.031, 24.0661)
  line L651 (181.031, 24.0661) -> (195.031, 24.0661)
  line L652 (195.031, 24.0661) -> (195.031, 25.0665)
  line L653 (195.031, 25.0665) -> (195.832, 25.0665)
  line L654 (195.832, 25.0665) -> (195.832, 28.1671)
  line L655 (195.832, 28.1671) -> (195.031, 28.1671)
  line L656 (195.031, 28.1671) -> (195.031, 33.9673)
  line L657 (195.031, 33.9673) -> (195.832, 33.9673)
  line L658 (195.832, 33.9673) -> (195.832, 37.0664)
  line L659 (195.832, 37.0664) -> (195.031, 37.0664)
  line L660 (195.031, 37.0664) -> (195.031, 38.0668)
  line L661 (195.031, 38.0668) -> (181.031, 38.0668)
  line L662 (200.081, 38.0668) -> (200.081, 37.0664)
  line L663 (200.081, 37.0664) -> (199.281, 37.0664)
  line L664 (199.281, 37.0664) -> (199.281, 33.9673)
  line L665 (199.281, 33.9673) -> (200.081, 33.9673)
  line L666 (200.081, 33.9673) -> (200.081, 28.1671)
  line L667 (200.081, 28.1671) -> (199.281, 28.1671)
  line L668 (199.281, 28.1671) -> (199.281, 25.0665)
  line L669 (199.281, 25.0665) -> (200.081, 25.0665)
  line L670 (200.081, 25.0665) -> (200.081, 24.0661)
  line L671 (200.081, 24.0661) -> (214.081, 24.0661)
  line L672 (214.081, 24.0661) -> (214.081, 25.0665)
  line L673 (214.081, 25.0665) -> (214.882, 25.0665)
  line L674 (214.882, 25.0665) -> (214.882, 28.1671)
  line L675 (214.882, 28.1671) -> (214.081, 28.1671)
  line L676 (214.081, 28.1671) -> (214.081, 33.9673)
  line L677 (214.081, 33.9673) -> (214.882, 33.9673)
  line L678 (214.882, 33.9673) -> (214.882, 37.0664)
  line L679 (214.882, 37.0664) -> (214.081, 37.0664)
  line L680 (214.081, 37.0664) -> (214.081, 38.0668)
  line L681 (214.081, 38.0668) -> (200.081, 38.0668)
  line L682 (219.131, 38.0668) -> (219.131, 37.0664)
  line L683 (219.131, 37.0664) -> (218.331, 37.0664)
  line L684 (218.331, 37.0664) -> (218.331, 33.9673)
  line L685 (218.331, 33.9673) -> (219.131, 33.9673)
  line L686 (219.131, 33.9673) -> (219.131, 28.1671)
  line L687 (219.131, 28.1671) -> (218.331, 28.1671)
  line L688 (218.331, 28.1671) -> (218.331, 25.0665)
  line L689 (218.331, 25.0665) -> (219.131, 25.0665)
  line L690 (219.131, 25.0665) -> (219.131, 24.0661)
  line L691 (219.131, 24.0661) -> (233.131, 24.0661)
  line L692 (233.131, 24.0661) -> (233.131, 25.0665)
  line L693 (233.131, 25.0665) -> (233.932, 25.0665)
  line L694 (233.932, 25.0665) -> (233.932, 28.1671)
  line L695 (233.932, 28.1671) -> (233.131, 28.1671)
  line L696 (233.131, 28.1671) -> (233.131, 33.9673)
  line L697 (233.131, 33.9673) -> (233.932, 33.9673)
  line L698 (233.932, 33.9673) -> (233.932, 37.0664)
  line L699 (233.932, 37.0664) -> (233.131, 37.0664)
  line L700 (233.131, 37.0664) -> (233.131, 38.0668)
  line L701 (233.131, 38.0668) -> (219.131, 38.0668)
  line L702 (314.381, 38.0668) -> (314.381, 37.0664)
  line L703 (314.381, 37.0664) -> (313.581, 37.0664)
  line L704 (313.581, 37.0664) -> (313.581, 33.9673)
  line L705 (313.581, 33.9673) -> (314.381, 33.9673)
  line L706 (314.381, 33.9673) -> (314.381, 28.1671)
  line L707 (314.381, 28.1671) -> (313.581, 28.1671)
  line L708 (313.581, 28.1671) -> (313.581, 25.0665)
  line L709 (313.581, 25.0665) -> (314.381, 25.0665)
  line L710 (314.381, 25.0665) -> (314.381, 24.0661)
  line L711 (314.381, 24.0661) -> (328.381, 24.0661)
  line L712 (328.381, 24.0661) -> (328.381, 25.0665)
  line L713 (328.381, 25.0665) -> (329.182, 25.0665)
  line L714 (329.182, 25.0665) -> (329.182, 28.1671)
  line L715 (329.182, 28.1671) -> (328.381, 28.1671)
  line L716 (328.381, 28.1671) -> (328.381, 33.9673)
  line L717 (328.381, 33.9673) -> (329.182, 33.9673)
  line L718 (329.182, 33.9673) -> (329.182, 37.0664)
  line L719 (329.182, 37.0664) -> (328.381, 37.0664)
  line L720 (328.381, 37.0664) -> (328.381, 38.0668)
  line L721 (328.381, 38.0668) -> (314.381, 38.0668)
  line L722 (357.244, 38.0668) -> (357.244, 37.0664)
  line L723 (357.244, 37.0664) -> (356.443, 37.0664)
  line L724 (356.443, 37.0664) -> (356.443, 33.9673)
  line L725 (356.443, 33.9673) -> (357.244, 33.9673)
  line L726 (357.244, 33.9673) -> (357.244, 28.1671)
  line L727 (357.244, 28.1671) -> (356.443, 28.1671)
  line L728 (356.443, 28.1671) -> (356.443, 25.0665)
  line L729 (356.443, 25.0665) -> (357.244, 25.0665)
  line L730 (357.244, 25.0665) -> (357.244, 24.0661)
  line L731 (357.244, 24.0661) -> (371.246, 24.0661)
  line L732 (371.246, 24.0661) -> (371.246, 25.0665)
  line L733 (371.246, 25.0665) -> (372.043, 25.0665)
  line L734 (372.043, 25.0665) -> (372.043, 28.1671)
  line L735 (372.043, 28.1671) -> (371.246, 28.1671)
  line L736 (371.246, 28.1671) -> (371.246, 33.9673)
  line L737 (371.246, 33.9673) -> (372.043, 33.9673)
  line L738 (372.043, 33.9673) -> (372.043, 37.0664)
  line L739 (372.043, 37.0664) -> (371.246, 37.0664)
  line L740 (371.246, 37.0664) -> (371.246, 38.0668)
  line L741 (371.246, 38.0668) -> (357.244, 38.0668)
  line L742 (376.294, 38.0668) -> (376.294, 37.0664)
  line L743 (376.294, 37.0664) -> (375.493, 37.0664)
  line L744 (375.493, 37.0664) -> (375.493, 33.9673)
  line L745 (375.493, 33.9673) -> (376.294, 33.9673)
  line L746 (376.294, 33.9673) -> (376.294, 28.1671)
  line L747 (376.294, 28.1671) -> (375.493, 28.1671)
  line L748 (375.493, 28.1671) -> (375.493, 25.0665)
  line L749 (375.493, 25.0665) -> (376.294, 25.0665)
  line L750 (376.294, 25.0665) -> (376.294, 24.0661)
  line L751 (376.294, 24.0661) -> (390.296, 24.0661)
  line L752 (390.296, 24.0661) -> (390.296, 25.0665)
  line L753 (390.296, 25.0665) -> (391.093, 25.0665)
  line L754 (391.093, 25.0665) -> (391.093, 28.1671)
  line L755 (391.093, 28.1671) -> (390.296, 28.1671)
  line L756 (390.296, 28.1671) -> (390.296, 33.9673)
  line L757 (390.296, 33.9673) -> (391.093, 33.9673)
  line L758 (391.093, 33.9673) -> (391.093, 37.0664)
  line L759 (391.093, 37.0664) -> (390.296, 37.0664)
  line L760 (390.296, 37.0664) -> (390.296, 38.0668)
  line L761 (390.296, 38.0668) -> (376.294, 38.0668)
  line L762 (395.344, 38.0668) -> (395.344, 37.0664)
  line L763 (395.344, 37.0664) -> (394.543, 37.0664)
  line L764 (394.543, 37.0664) -> (394.543, 33.9673)
  line L765 (394.543, 33.9673) -> (395.344, 33.9673)
  line L766 (395.344, 33.9673) -> (395.344, 28.1671)
  line L767 (395.344, 28.1671) -> (394.543, 28.1671)
  line L768 (394.543, 28.1671) -> (394.543, 25.0665)
  line L769 (394.543, 25.0665) -> (395.344, 25.0665)
  line L770 (395.344, 25.0665) -> (395.344, 24.0661)
  line L771 (395.344, 24.0661) -> (409.346, 24.0661)
  line L772 (409.346, 24.0661) -> (409.346, 25.0665)
  line L773 (409.346, 25.0665) -> (410.143, 25.0665)
  line L774 (410.143, 25.0665) -> (410.143, 28.1671)
  line L775 (410.143, 28.1671) -> (409.346, 28.1671)
  line L776 (409.346, 28.1671) -> (409.346, 33.9673)
  line L777 (409.346, 33.9673) -> (410.143, 33.9673)
  line L778 (410.143, 33.9673) -> (410.143, 37.0664)
  line L779 (410.143, 37.0664) -> (409.346, 37.0664)
  line L780 (409.346, 37.0664) -> (409.346, 38.0668)
  line L781 (409.346, 38.0668) -> (395.344, 38.0668)
  line L782 (11.9628, 57.1168) -> (11.9628, 56.1164)
  line L783 (11.9628, 56.1164) -> (11.1621, 56.1164)
  line L784 (11.1621, 56.1164) -> (11.1621, 53.0172)
  line L785 (11.1621, 53.0172) -> (11.9628, 53.0172)
  line L786 (11.9628, 53.0172) -> (11.9628, 47.2172)
  line L787 (11.9628, 47.2172) -> (11.1621, 47.2172)
  line L788 (11.1621, 47.2172) -> (11.1621, 44.1166)
  line L789 (11.1621, 44.1166) -> (11.9628, 44.1166)
  line L790 (11.9628, 44.1166) -> (11.9628, 43.1161)
  line L791 (11.9628, 43.1161) -> (25.9623, 43.1161)
  line L792 (25.9623, 43.1161) -> (25.9623, 44.1166)
  line L793 (25.9623, 44.1166) -> (26.7629, 44.1166)
  line L794 (26.7629, 44.1166) -> (26.7629, 47.2172)
  line L795 (26.7629, 47.2172) -> (25.9623, 47.2172)
  line L796 (25.9623, 47.2172) -> (25.9623, 53.0172)
  line L797 (25.9623, 53.0172) -> (26.7629, 53.0172)
  line L798 (26.7629, 53.0172) -> (26.7629, 56.1164)
  line L799 (26.7629, 56.1164) -> (25.9623, 56.1164)
  line L800 (25.9623, 56.1164) -> (25.9623, 57.1168)
  line L801 (25.9623, 57.1168) -> (11.9628, 57.1168)
  line L802 (38.1564, 57.1168) -> (38.1564, 56.1164)
  line L803 (38.1564, 56.1164) -> (37.356, 56.1164)
  line L804 (37.356, 56.1164) -> (37.356, 53.0172)
  line L805 (37.356, 53.0172) -> (38.1564, 53.0172)
  line L806 (38.1564, 53.0172) -> (38.1564, 47.2172)
  line L807 (38.1564, 47.2172) -> (37.356, 47.2172)
  line L808 (37.356, 47.2172) -> (37.356, 44.1166)
  line L809 (37.356, 44.1166) -> (38.1564, 44.1166)
  line L810 (38.1564, 44.1166) -> (38.1564, 43.1161)
  line L811 (38.1564, 43.1161) -> (52.1561, 43.1161)
  line L812 (52.1561, 43.1161) -> (52.1561, 44.1166)
  line L813 (52.1561, 44.1166) -> (52.9565, 44.1166)
  line L814 (52.9565, 44.1166) -> (52.9565, 47.2172)
  line L815 (52.9565, 47.2172) -> (52.1561, 47.2172)
  line L816 (52.1561, 47.2172) -> (52.1561, 53.0172)
  line L817 (52.1561, 53.0172) -> (52.9565, 53.0172)
  line L818 (52.9565, 53.0172) -> (52.9565, 56.1164)
  line L819 (52.9565, 56.1164) -> (52.1561, 56.1164)
  line L820 (52.1561, 56.1164) -> (52.1561, 57.1168)
  line L821 (52.1561, 57.1168) -> (38.1564, 57.1168)
  line L822 (57.2064, 57.1168) -> (57.2064, 56.1164)
  line L823 (57.2064, 56.1164) -> (56.406, 56.1164)
  line L824 (56.406, 56.1164) -> (56.406, 53.0172)
  line L825 (56.406, 53.0172) -> (57.2064, 53.0172)
  line L826 (57.2064, 53.0172) -> (57.2064, 47.2172)
  line L827 (57.2064, 47.2172) -> (56.406, 47.2172)
  line L828 (56.406, 47.2172) -> (56.406, 44.1166)
  line L829 (56.406, 44.1166) -> (57.2064, 44.1166)
  line L830 (57.2064, 44.1166) -> (57.2064, 43.1161)
  line L831 (57.2064, 43.1161) -> (71.2061, 43.1161)
  line L832 (71.2061, 43.1161) -> (71.2061, 44.1166)
  line L833 (71.2061, 44.1166) -> (72.0065, 44.1166)
  line L834 (72.0065, 44.1166) -> (72.0065, 47.2172)
  line L835 (72.0065, 47.2172) -> (71.2061, 47.2172)
  line L836 (71.2061, 47.2172) -> (71.2061, 53.0172)
  line L837 (71.2061, 53.0172) -> (72.0065, 53.0172)
  line L838 (72.0065, 53.0172) -> (72.0065, 56.1164)
  line L839 (72.0065, 56.1164) -> (71.2061, 56.1164)
  line L840 (71.2061, 56.1164) -> (71.2061, 57.1168)
  line L841 (71.2061, 57.1168) -> (57.2064, 57.1168)
  line L842 (76.2564, 57.1168) -> (76.2564, 56.1164)
  line L843 (76.2564, 56.1164) -> (75.456, 56.1164)
  line L844 (75.456, 56.1164) -> (75.456, 53.0172)
  line L845 (75.456, 53.0172) -> (76.2564, 53.0172)
  line L846 (76.2564, 53.0172) -> (76.2564, 47.2172)
  line L847 (76.2564, 47.2172) -> (75.456, 47.2172)
  line L848 (75.456, 47.2172) -> (75.456, 44.1166)
  line L849 (75.456, 44.1166) -> (76.2564, 44.1166)
  line L850 (76.2564, 44.1166) -> (76.2564, 43.1161)
  line L851 (76.2564, 43.1161) -> (90.2561, 43.1161)
  line L852 (90.2561, 43.1161) -> (90.2561, 44.1166)
  line L853 (90.2561, 44.1166) -> (91.0565, 44.1166)
  line L854 (91.0565, 44.1166) -> (91.0565, 47.2172)
  line L855 (91.0565, 47.2172) -> (90.2561, 47.2172)
  line L856 (90.2561, 47.2172) -> (90.2561, 53.0172)
  line L857 (90.2561, 53.0172) -> (91.0565, 53.0172)
  line L858 (91.0565, 53.0172) -> (91.0565, 56.1164)
  line L859 (91.0565, 56.1164) -> (90.2561, 56.1164)
  line L860 (90.2561, 56.1164) -> (90.2561, 57.1168)
  line L861 (90.2561, 57.1168) -> (76.2564, 57.1168)
  line L862 (95.3064, 57.1168) -> (95.3064, 56.1164)
  line L863 (95.3064, 56.1164) -> (94.506, 56.1164)
  line L864 (94.506, 56.1164) -> (94.506, 53.0172)
  line L865 (94.506, 53.0172) -> (95.3064, 53.0172)
  line L866 (95.3064, 53.0172) -> (95.3064, 47.2172)
  line L867 (95.3064, 47.2172) -> (94.506, 47.2172)
  line L868 (94.506, 47.2172) -> (94.506, 44.1166)
  line L869 (94.506, 44.1166) -> (95.3064, 44.1166)
  line L870 (95.3064, 44.1166) -> (95.3064, 43.1161)
  line L871 (95.3064, 43.1161) -> (109.306, 43.1161)
  line L872 (109.306, 43.1161) -> (109.306, 44.1166)
  line L873 (109.306, 44.1166) -> (110.107, 44.1166)
  line L874 (110.107, 44.1166) -> (110.107, 47.2172)
  line L875 (110.107, 47.2172) -> (109.306, 47.2172)
  line L876 (109.306, 47.2172) -> (109.306, 53.0172)
  line L877 (109.306, 53.0172) -> (110.107, 53.0172)
  line L878 (110.107, 53.0172) -> (110.107, 56.1164)
  line L879 (110.107, 56.1164) -> (109.306, 56.1164)
  line L880 (109.306, 56.1164) -> (109.306, 57.1168)
  line L881 (109.306, 57.1168) -> (95.3064, 57.1168)
  line L882 (114.356, 57.1168) -> (114.356, 56.1164)
  line L883 (114.356, 56.1164) -> (113.556, 56.1164)
  line L884 (113.556, 56.1164) -> (113.556, 53.0172)
  line L885 (113.556, 53.0172) -> (114.356, 53.0172)
  line L886 (114.356, 53.0172) -> (114.356, 47.2172)
  line L887 (114.356, 47.2172) -> (113.556, 47.2172)
  line L888 (113.556, 47.2172) -> (113.556, 44.1166)
  line L889 (113.556, 44.1166) -> (114.356, 44.1166)
  line L890 (114.356, 44.1166) -> (114.356, 43.1161)
  line L891 (114.356, 43.1161) -> (128.356, 43.1161)
  line L892 (128.356, 43.1161) -> (128.356, 44.1166)
  line L893 (128.356, 44.1166) -> (129.157, 44.1166)
  line L894 (129.157, 44.1166) -> (129.157, 47.2172)
  line L895 (129.157, 47.2172) -> (128.356, 47.2172)
  line L896 (128.356, 47.2172) -> (128.356, 53.0172)
  line L897 (128.356, 53.0172) -> (129.157, 53.0172)
  line L898 (129.157, 53.0172) -> (129.157, 56.1164)
  line L899 (129.157, 56.1164) -> (128.356, 56.1164)
  line L900 (128.356, 56.1164) -> (128.356, 57.1168)
  line L901 (128.356, 57.1168) -> (114.356, 57.1168)
  line L902 (133.406, 57.1168) -> (133.406, 56.1164)
  line L903 (133.406, 56.1164) -> (132.606, 56.1164)
  line L904 (132.606, 56.1164) -> (132.606, 53.0172)
  line L905 (132.606, 53.0172) -> (133.406, 53.0172)
  line L906 (133.406, 53.0172) -> (133.406, 47.2172)
  line L907 (133.406, 47.2172) -> (132.606, 47.2172)
  line L908 (132.606, 47.2172) -> (132.606, 44.1166)
  line L909 (132.606, 44.1166) -> (133.406, 44.1166)
  line L910 (133.406, 44.1166) -> (133.406, 43.1161)
  line L911 (133.406, 43.1161) -> (147.406, 43.1161)
  line L912 (147.406, 43.1161) -> (147.406, 44.1166)
  line L913 (147.406, 44.1166) -> (148.207, 44.1166)
  line L914 (148.207, 44.1166) -> (148.207, 47.2172)
  line L915 (148.207, 47.2172) -> (147.406, 47.2172)
  line L916 (147.406, 47.2172) -> (147.406, 53.0172)
  line L917 (147.406, 53.0172) -> (148.207, 53.0172)
  line L918 (148.207, 53.0172) -> (148.207, 56.1164)
  line L919 (148.207, 56.1164) -> (147.406, 56.1164)
  line L920 (147.406, 56.1164) -> (147.406, 57.1168)
  line L921 (147.406, 57.1168) -> (133.406, 57.1168)
  line L922 (152.456, 57.1168) -> (152.456, 56.1164)
  line L923 (152.456, 56.1164) -> (151.656, 56.1164)
  line L924 (151.656, 56.1164) -> (151.656, 53.0172)
  line L925 (151.656, 53.0172) -> (152.456, 53.0172)
  line L926 (152.456, 53.0172) -> (152.456, 47.2172)
  line L927 (152.456, 47.2172) -> (151.656, 47.2172)
  line L928 (151.656, 47.2172) -> (151.656, 44.1166)
  line L929 (151.656, 44.1166) -> (152.456, 44.1166)
  line L930 (152.456, 44.1166) -> (152.456, 43.1161)
  line L931 (152.456, 43.1161) -> (166.456, 43.1161)
  line L932 (166.456, 43.1161) -> (166.456, 44.1166)
  line L933 (166.456, 44.1166) -> (167.257, 44.1166)
  line L934 (167.257, 44.1166) -> (167.257, 47.2172)
  line L935 (167.257, 47.2172) -> (166.456, 47.2172)
  line L936 (166.456, 47.2172) -> (166.456, 53.0172)
  line L937 (166.456, 53.0172) -> (167.257, 53.0172)
  line L938 (167.257, 53.0172) -> (167.257, 56.1164)
  line L939 (167.257, 56.1164) -> (166.456, 56.1164)
  line L940 (166.456, 56.1164) -> (166.456, 57.1168)
  line L941 (166.456, 57.1168) -> (152.456, 57.1168)
  line L942 (171.506, 57.1168) -> (171.506, 56.1164)
  line L943 (171.506, 56.1164) -> (170.706, 56.1164)
  line L944 (170.706, 56.1164) -> (170.706, 53.0172)
  line L945 (170.706, 53.0172) -> (171.506, 53.0172)
  line L946 (171.506, 53.0172) -> (171.506, 47.2172)
  line L947 (171.506, 47.2172) -> (170.706, 47.2172)
  line L948 (170.706, 47.2172) -> (170.706, 44.1166)
  line L949 (170.706, 44.1166) -> (171.506, 44.1166)